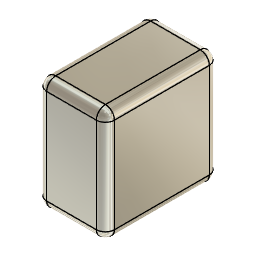
5x5x3 (Autodesk Fusion 360 design; units mm, degrees)
Autodesk Fusion 360 part; units mm, degrees
sketch "Sketch1" plane through (0, 0, 0) normal (0, 0, 1) x (1, 0, 0)
  line L0 (1.5, -2.5) -> (-1.5, -2.5)
  line L1 (-1.5, -2.5) -> (-1.5, 2.5)
  line L2 (-1.5, 2.5) -> (1.5, 2.5)
  line L3 (1.5, 2.5) -> (1.5, -2.5)
  line L4 (1.5, -2.5) -> (-1.5, 2.5) construction
  line L5 (-1.5, -2.5) -> (1.5, 2.5) construction
  dimension "d1" = 3
  dimension "d2" = 5
  constraint horizontal L0
  constraint perpendicular L0 L1
  constraint parallel L0 L2
  constraint parallel L1 L3
  constraint coincident L4 origin
  constraint coincident L5 origin
  measures "d1" distance of L1.end L2.end
  measures "d2" distance of L0.end L1.end
extrude "Extrude1" add sketch "Sketch1" along normal blind 5
fillet "Fillet1" radius 0.4 6 faces at (0.5, -0.8333, 5) (0.5, -2.5, 1.6667) (1.5, 0.8333, 1.6667) (-1.5, -0.8333, 1.6667) (-0.5, 2.5, 1.6667) (0.5, -0.8333, 0)
named bodies: "5x5x3"
